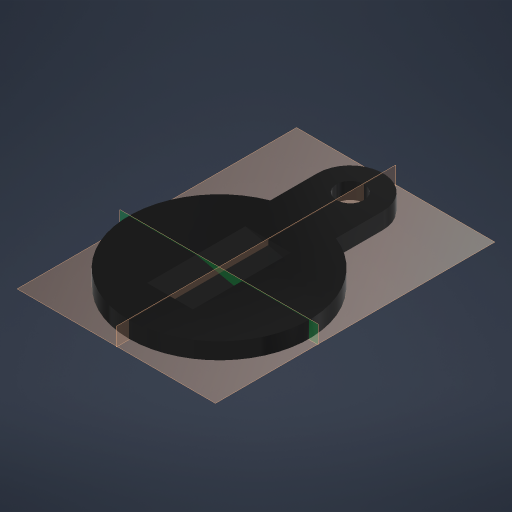
# Autodesk Inventor part: Filler Cap
Saved by Autodesk Inventor 2024 (Build 280153000, 153)
## iProperties
Manager: Louis Van Roosmaelen
Company: DCS - DIGITAL COMBAT SIMULATOR
Created: 2023-11-03
Part Number: Filler Cap
Material: S235
Catalog Web Link: http://emmausbovenbouw.op-weg.be/
Vendor: Emmaüsinstituut Bovenbouw Aalter
Document SubType Name: Modeling
Designer: Louis
Engineer: Declercq St.
Manufacturer: Standard
Standards Organization: Custom
Density: 7.86 g/cm^3
Appearance: Smooth - Black
IDENT.NR.: AJ2022
TEAM: 30
Title: F18C Home Cockpit
Author: Louis
Keywords: Ø
Autodesk Inventor part; units mm, degrees
sketch "Sketch1" plane through (0, 0, 0) normal (0, 0, 1) x (1, 0, 0)
  line L0 (0, 2.8582) -> (0, -2.8582) construction
  line L1 (-5.7775, 0) -> (5.7775, 0) construction
  circle A0 centre (0, 0) radius 13.75
  line L2 (5, 12.8087) -> (5, 25)
  line L3 (5, 25) -> (-5, 25)
  line L4 (-5, 25) -> (-5, 12.8087)
  line L5 (0, 32.75) -> (0, -21.5) construction
  point P0 (0, 20)
  dimension "d0" = 27.5
  dimension "d1" = 20
  dimension "d2" = 5
  dimension "d3" = 5
  dimension "d4" = 5
  constraints: 10 end point, 2 coincident, 2 midpoint, 2 perpendicular, 2 point on circle, 2 vertical, 1 centre point, 1 horizontal, 1 point on line
  measures "d0" diameter of A0
  measures "d1" distance of point (0, 0) point (0, 20)
  measures "d2" distance between parallel lines of L5 L4
  measures "d3" distance from line of point (0, 20) L3
  measures "d4" distance from line of point (0, 20) L2
extrude "Extrusion1" add sketch "Sketch1" along normal blind 2.5
sketch "Sketch2" plane through (0, 0, 2.5) normal (0, 0, 1) x (1, 0, 0)
  line L0 (-5, 25) -> (-5, 12.8087) projected
  arc A0 (-5, 12.8087) -> (5, 12.8087) centre (0, 0) ccw projected
  line L1 (-5, 12.8087) -> (-5, 25) projected
  line L2 (-5, 25) -> (5, 25) projected
  line L3 (5, 25) -> (5, 12.8087) projected
  point P0 (0, 20)
  dimension "d7" = 5
  dimension "d8" = 5
  measures "d7" distance from line of L0 point (0, 20)
  measures "d8" distance from line of L2 point (0, 20)
hole "Hole1" at (0, 20, 2.5) direction (0, 0, -1) diameter 4.2 end through all
fillet "Fillet1" radius 5 2 edges at (-5, 25, 1.25) (5, 25, 1.25)
sketch "Sketch3" plane through (0, 0, 0) normal (1, 0, 0) x (0, 1, 0)
  line L0 (12.8087, 2.5) -> (-13.75, 2.5) projected
  line L1 (-7.5, 2.5) -> (7.5, 2.5)
  line L2 (7.5, 2.5) -> (7.5, 1)
  line L3 (7.5, 1) -> (-7.5, 1)
  line L4 (-7.5, 1) -> (-7.5, 2.5)
  line L5 (0, 3) -> (0, -0.5) projected
  line L6 (22.1, 2.5) -> (25, 2.5) projected
  line L7 (25, 2.5) -> (25, 0) projected
  line L8 (25, 0) -> (22.1, 0) projected
  line L9 (22.1, 0) -> (22.1, 2.5) projected
  line L10 (17.9, 0) -> (-13.75, 0) projected
  line L11 (-13.75, 0) -> (-13.75, 2.5) projected
  line L12 (-13.75, 2.5) -> (17.9, 2.5) projected
  line L13 (17.9, 2.5) -> (17.9, 0) projected
  point P0 (0, 0)
  point P1 (7.5, 2.5)
  dimension "d17" = 15
  dimension "d18" = 7.5
  dimension "d19" = 1.5
  constraints: 8 end point, 2 parallel, 1 horizontal, 1 perpendicular, 1 point on line
  measures "d17" distance of L2.end L3.end
  measures "d18" distance between parallel lines of L5 L4
  measures "d19" distance between parallel lines of L0 L3
extrude "Extrusion2" cut sketch "Sketch3" along normal mid plane 7 contours L2 L3 L5 L0 | L5 L3 L4 L0
sketch "Sketch4" plane through (-3.5, 7.5, 2.5) normal (0, -1, 0) x (1, 0, 0)
  line L0 (15.0244, -2.5) -> (-8.0244, -2.5) projected
  line L1 (-8.0244, -2.5) -> (-8.0244, 0) projected
  line L2 (-8.0244, 0) -> (0, 0) projected
  line L3 (0, 0) -> (7, 0) projected
  line L4 (7, 0) -> (7, -1.5) projected
  line L5 (7, -1.5) -> (0, -1.5) projected
  line L6 (0, 0) -> (0, -1.5) projected
  line L7 (15.0244, 0) -> (15.0244, -2.5) projected
  line L8 (7, 0) -> (15.0244, 0) projected
  line L9 (0, 0) -> (7, -1.5)
  point P0 (3.5, -2.5)
  constraints: 2 end point
extrude "Extrusion3" add sketch "Sketch4" along normal up to surface (15 mm away) contours L9 L5 L6
equation "\"d18\" = 0.5 * d17"
body "Solid1"
